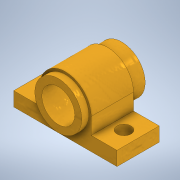
# Autodesk Inventor part: Part11
Saved by Autodesk Inventor 2020 (Build 240168000, 168)
## iProperties
Created: 2021-10-14
Part Number: Part11
Material: Brass, Soft Yellow, Welded
Document SubType Name: Modeling
Designer: simon.erikssonwestl
Density: 8.5 g/cm^3
Appearance: Weld - Brass
Author: simon.erikssonwestl
Autodesk Inventor part; units mm, degrees
ref_plane "YZ Plane" through (0, 0, 0) normal (1, 0, 0) x (0, 1, 0)
ref_plane "XZ Plane" through (0, 0, 0) normal (0, 1, 0) x (-1, 0, 0)
ref_plane "XY Plane" through (0, 0, 0) normal (0, 0, 1) x (1, 0, 0)
sketch "Sketch1" plane through (0, 0, 0) normal (0, 1, 0) x (-1, 0, 0)
  line L0 (11, -4.5) -> (-11, -4.5)
  line L1 (-11, -4.5) -> (-11, 4.5)
  line L2 (-11, 4.5) -> (11, 4.5)
  line L3 (11, 4.5) -> (11, -4.5)
  line L4 (11, -4.5) -> (-11, 4.5) construction
  line L5 (-11, -4.5) -> (11, 4.5) construction
  point P0 (0, 0)
  dimension "d0" = 22
  dimension "d1" = 9
  constraints: 12 end point, 2 midpoint, 2 parallel, 1 horizontal, 1 perpendicular
  measures "d0" distance of L1.end L2.end
  measures "d1" distance of L0.end L1.end
extrude "Extrusion1" add sketch "Sketch1" along normal mid plane 3
sketch "Sketch2" plane through (-11, 1.5, 4.5) normal (0, 0, 1) x (1, 0, 0)
  line L0 (11, 9) -> (11, 9)
  line L1 (16.5, 3.5) -> (16.5, 0)
  line L2 (16.5, 0) -> (5.5, 0)
  line L3 (5.5, 0) -> (5.5, 3.5)
  line L4 (22, 0) -> (0, 0) projected
  line L5 (5.5, 4.5) -> (16.5, -4.5) construction
  line L6 (16.5, 4.5) -> (5.5, -4.5) construction
  arc A0 (11, 9) -> (5.5, 3.5) centre (11, 3.5) ccw
  arc A1 (16.5, 3.5) -> (11, 9) centre (11, 3.5) ccw
  point P0 (11, -1.5)
  point P1 (16.5, 9)
  point P2 (11, 0)
  dimension "d4" = 11
  dimension "d5" = 9
  dimension "d6" = 0
  dimension "d7" = 5.5
  constraints: 12 end point, 4 point on circle, 4 tangent, 3 midpoint, 2 centre point, 2 parallel, 2 point on line, 1 concentric, 1 horizontal, 1 perpendicular
  measures "d4" distance of L1.end L2.end
  measures "d5" distance of point (16.5, 9) L1.end
  measures "d6" distance between parallel lines of L4 L2
  measures "d7" radius of A0
extrude "Extrusion2" add sketch "Sketch2" against normal blind 9
sketch "Sketch3" plane through (-11, -1.5, 4.5) normal (0, 0, 1) x (1, 0, 0)
  circle A0 centre (11, 6.5) radius 5
  line L0 (5.5, 6.5) -> (5.5, 3) projected
  point P0 (11, 1.5)
  dimension "d10" = 10
  dimension "d11" = 5.5
  constraints: 1 centre point
  measures "d10" diameter of A0
  measures "d11" distance from line of L0 A0.centre
extrude "Extrusion3" add sketch "Sketch3" along normal blind 1.5
sketch "Sketch4" plane through (11, -1.5, -4.5) normal (0, 0, -1) x (-1, 0, 0)
  arc A0 (16.5, 6.5) -> (5.5, 6.5) centre (11, 6.5) ccw projected
  circle A1 centre (11, 6.5) radius 5
  point P0 (11, 1.5)
  dimension "d14" = 10
  constraints: 1 centre point, 1 coincident
  measures "d14" diameter of A1
extrude "Extrusion4" add sketch "Sketch4" along normal blind 3
sketch "Sketch5" plane through (0, 5, -7.5) normal (0, 0, -1) x (-1, 0, 0)
  circle A0 centre (0, 0) radius 3.5
  point P0 (0, -5)
  dimension "d17" = 7
  constraints: 1 centre point
  measures "d17" diameter of A0
extrude "Extrusion5" cut sketch "Sketch5" against normal through all
sketch "Sketch6" plane through (0, -1.5, 0) normal (0, -1, 0) x (1, 0, 0)
  circle A0 centre (-8, 0) radius 1.5
  line L0 (-11, 4.5) -> (-11, -4.5) projected
  point P0 (0, 0)
  dimension "d20" = 3
  dimension "d21" = 3
  constraints: 1 centre point
  measures "d20" diameter of A0
  measures "d21" distance from line of L0 A0.centre
extrude "Extrusion6" cut sketch "Sketch6" against normal through all
sketch "Sketch7" plane through (0, -1.5, 0) normal (0, -1, 0) x (1, 0, 0)
  circle A0 centre (8, 0) radius 1.5
  line L0 (11, -4.5) -> (11, 4.5) projected
  point P0 (0, 0)
  dimension "d24" = 3
  dimension "d25" = 3
  constraints: 1 centre point
  measures "d24" diameter of A0
  measures "d25" distance from line of L0 A0.centre
extrude "Extrusion7" cut sketch "Sketch7" against normal through all
sketch "Sketch8" plane through (0, -1.5, 0) normal (0, -1, 0) x (1, 0, 0)
  circle A0 centre (0, 0) radius 1.5
  dimension "d28" = 3
  constraints: 1 centre point, 1 coincident
  measures "d28" diameter of A0
hole "Hole1" at (0, -1.5, 0) direction (0, 1, 0) diameter 1 depth 3.04 tip angle 118 countersink diameter 3 countersink angle 90
body "Solid1"
